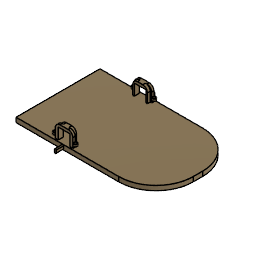
lab12 (Autodesk Fusion 360 design; units mm, degrees)
part number: 2026-05-18-18-22-44-675
Autodesk Fusion 360 part; units mm, degrees
sketch "sasiu" plane through (0, 0, 0) normal (0, 0, 1) x (1, 0, 0)
  line L0 (0, 0) -> (150, 0)
  line L1 (150, 0) -> (150, 90)
  line L2 (150, 90) -> (0, 90)
  line L3 (0, 90) -> (0, 0)
  line L4 (0, 0) -> (50, 0) construction
  line L5 (0, 0) -> (50, 0) construction
  line L6 (0, 90) -> (50, 90) construction
  line L7 (50, 0) -> (56.25, 0) construction
  line L8 (50, 0) -> (43.75, 0) construction
  line L9 (56.25, 0) -> (43.75, 0) construction
  line L10 (43.75, 0) -> (43.75, 24.2)
  line L11 (43.75, 24.2) -> (56.25, 24.2)
  line L12 (56.25, 24.2) -> (56.25, 0)
  line L13 (50, 90) -> (56.25, 90) construction
  line L14 (50, 90) -> (43.75, 90) construction
  line L15 (56.25, 90) -> (43.8642, 90) construction
  line L16 (43.8642, 90) -> (43.8642, 65.8)
  line L17 (43.8642, 65.8) -> (56.25, 65.8)
  line L18 (56.25, 65.8) -> (56.25, 90)
  line L19 (51, 0) -> (49, 0)
  line L20 (49, 0) -> (49, -7.85)
  line L21 (49, -7.85) -> (51, -7.85)
  line L22 (51, -7.85) -> (51, 0)
  line L23 (51, 90) -> (48.9753, 90)
  line L24 (48.9753, 90) -> (48.9753, 97.85)
  line L25 (48.9753, 97.85) -> (51, 97.85)
  line L26 (51, 97.85) -> (51, 90)
  line L27 (65.2982, 87.1869) -> (35.2982, 87.1869)
  line L28 (150, 45) -> (0, 45)
  line L29 (65.2982, 2.8131) -> (35.2982, 2.8131)
  line L30 (50, 90) -> (50, 0)
  circle A0 centre (60.9428, 87.1869) radius 2
  circle A1 centre (39.0572, 87.1869) radius 2
  circle A2 centre (60.9428, 2.8131) radius 2
  circle A3 centre (39.0572, 2.8131) radius 2
  circle A4 centre (60.9428, 87.1869) radius 1.25
  circle A5 centre (39.0572, 87.1869) radius 1.25
  circle A6 centre (60.9428, 2.8131) radius 1.25
  circle A7 centre (39.0572, 2.8131) radius 1.25
  line L31 (59.4051, 88.4658) -> (56.25, 88.4658)
  line L32 (56.25, 88.4658) -> (56.25, 85.9998)
  line L33 (56.25, 85.9998) -> (59.4051, 85.9998)
  line L34 (59.4051, 85.9998) -> (59.4051, 88.4658)
  line L35 (59.4051, 1.5342) -> (56.25, 1.5342)
  line L36 (59.4051, 4.0002) -> (59.4051, 1.5342)
  line L37 (56.25, 4.0002) -> (59.4051, 4.0002)
  line L38 (40.6669, 88.3739) -> (43.8642, 88.3739)
  line L39 (43.8642, 88.3739) -> (43.8642, 86)
  line L40 (43.8642, 86) -> (40.6669, 86)
  line L41 (40.6669, 86) -> (40.6669, 88.3739)
  line L42 (56.25, 88.4658) -> (43.8642, 88.4658)
  line L43 (57.8275, 85.9998) -> (57.8275, 83)
  line L44 (57.8275, 83) -> (42, 83)
  line L45 (42, 83) -> (42, 86)
  line L46 (57.8275, 7) -> (42, 7)
  line L47 (57.8275, 4.0002) -> (57.8275, 7)
  line L48 (42, 7) -> (42, 4)
  line L49 (43.75, 4.0002) -> (40.5949, 4.0002)
  line L50 (40.5949, 1.5342) -> (43.75, 1.5342)
  line L51 (40.5949, 4.0002) -> (40.5949, 1.5342)
  line L52 (56.25, 1.5342) -> (43.75, 1.5342)
  line L53 (57.8275, 85.9998) -> (57.8275, 88.4658)
  line L54 (42, 86) -> (42, 88.3739)
  line L55 (42, 4) -> (42, 1.5342)
  line L56 (57.8275, 4.0002) -> (57.8275, 1.5342)
  dimension "d1" = 150
  dimension "d2" = 90
  dimension "d3" = 50
  dimension "d4" = 50
  dimension "d5" = 6.25
  dimension "d6" = 6.25
  dimension "d7" = 24.2
  dimension "d8" = 6.25
  dimension "d9" = 6.25
  dimension "d10" = 24.2
  dimension "d11" = 7.85
  dimension "d12" = 7.85
  dimension "d13" = 43.8642
  dimension "d14" = 43.75
  dimension "d15" = 2
  dimension "d16" = 48.9753
  dimension "d17" = 2.0247
  dimension "d18" = 49
  dimension "d21" = 4
  dimension "d22" = 2.5
  dimension "d29" = 2.3739
  dimension "d30" = 3.1974
  dimension "d31" = 2.466
  dimension "d32" = 18.8102
  dimension "d33" = 15.8275
  dimension "d34" = 30
  dimension "d35" = 35.2982
  dimension "d36" = 86
  dimension "d37" = 83
  constraint horizontal L0
  constraint vertical L1
  constraint horizontal L2
  constraint vertical L3
  constraint coincident L0.start L3.end
  constraint coincident L0 L4.end
  constraint perpendicular L3 L5
  constraint perpendicular L3 L6
  constraint parallel L0 L7
  constraint parallel L0 L8
  constraint horizontal L9
  constraint vertical L10
  constraint horizontal L11
  constraint vertical L12
  constraint parallel L2 L13
  constraint parallel L6 L14
  constraint horizontal L15
  constraint vertical L16
  constraint horizontal L17
  constraint vertical L18
  constraint horizontal L19
  constraint vertical L20
  constraint horizontal L21
  constraint vertical L22
  constraint coincident L9 L19.start
  constraint horizontal L23
  constraint vertical L24
  constraint horizontal L25
  constraint vertical L26
  constraint coincident L2 L23.start
  constraint perpendicular L16 L27
  constraint midpoint L1 L28.start
  constraint midpoint L3 L28.end
  constraint symmetric L27.start L28 L29.start
  constraint symmetric L27.end L28 L29.end
  constraint perpendicular L4 L30
  constraint coincident L27 A0.centre
  constraint symmetric L30 A0 A1
  constraint symmetric L28 A0 A2
  constraint symmetric L28 A1 A3
  constraint concentric A0 A4
  constraint symmetric L30 A4 A5
  constraint symmetric L28 A4 A6
  constraint symmetric L28 A5 A7
  constraint horizontal L31
  constraint vertical L32
  constraint horizontal L33
  constraint vertical L34
  constraint coincident L18 L32.end
  constraint coincident A0 L31.start
  constraint symmetric L28 L31.start L35.start
  constraint symmetric L28 L31.end L35.end
  constraint symmetric L28 L32.end L37.start
  constraint symmetric L28 L33.end L36.start
  constraint horizontal L38
  constraint vertical L39
  constraint horizontal L40
  constraint vertical L41
  constraint coincident L16 L39.end
  constraint coincident A1 L38.start
  constraint coincident A1 L40.end
  constraint coincident L16 L42.end
  constraint perpendicular L16 L42
  constraint midpoint L33 L43.start
  constraint perpendicular L33 L43
  constraint perpendicular L16 L44
  constraint coincident L40 L45.end
  constraint perpendicular L40 L45
  constraint symmetric L28 L43.start L47.start
  constraint symmetric L28 L43.end L46.start
  constraint symmetric L28 L44.end L46.end
  constraint symmetric L28 L45.end L48.end
  constraint symmetric L30 L35.start L50.start
  constraint symmetric L30 L35.end L50.end
  constraint symmetric L30 L36.start L49.end
  constraint symmetric L30 L37.start L49.start
  constraint midpoint L31 L53.end
  constraint coincident L38 L54.end
  constraint perpendicular L38 L54
  constraint coincident L50 L55.end
  constraint perpendicular L50 L55
  constraint midpoint L35 L56.end
  measures "d1" distance of L0.start L0.end
  measures "d2" distance of L0.start L2.end
  measures "d3" distance of L0.start L4.end
  measures "d4" distance of L2.end L6.end
  measures "d5" distance of L4.end L7.end
  measures "d6" distance of L4.end L8.end
  measures "d7" distance of L7.end L11.end
  measures "d8" distance of L6.end L13.end
  measures "d9" distance of L6.end L14.end
  measures "d10" distance of L13.end L17.end
  measures "d11" distance of L19.start L21.end
  measures "d12" distance of L23.start L25.end
  measures "d13" distance of L3 L16
  measures "d14" distance of L3 L10
  measures "d15" distance of L20 L22
  measures "d16" distance of L3 L24
  measures "d17" distance of L24 L26
  measures "d18" distance of L3 L20
  measures "d21" diameter of A0
  measures "d22" diameter of A4
  measures "d29" distance of L38 L40
  measures "d30" distance of L39 L41
  measures "d31" distance of L33 L42
  measures "d32" distance of L34 L51
  measures "d33" distance of L53 L54
  measures "d34" horizontal distance of L29.start L29.end
  measures "d35" distance of L3 L27.end
  measures "d36" distance of L0 L40
  measures "d37" distance of L0 L44
extrude "Extrude1" add sketch "sasiu" along normal blind 5 makes body 1
extrude "Extrude2" add sketch "sasiu" along normal blind 2 from surface at 8 separate body contours L29 A3 A7 L51 | L29 A3 A7 L49 L51 | L29 A2 A6 L36 | L29 A2 A6 L36 L37 | L27 A1 A5 L41 | L27 A1 A5 L41 | L27 A0 A4 L34 | L27 A0 A4 L33 L34 makes body 2 at (60.1621, 4.6544, 8.6667) makes body 3 at (38.8689, 0.8219, 8.6667) makes body 4 at (62.738, 88.0687, 9.3333) makes body 5 at (40.5426, 85.8478, 8.6667)
extrude "Extrude3" add sketch "sasiu" along normal blind 15 from surface at 5 contours L10 L29 L50 L55 | L10 L29 L49 L55 | L29 A3 L50 L55 | L10 L46 L48 L49 | L29 A3 L49 L55 | L29 A3 L51 | L12 L29 L35 L56 | L12 L29 L37 L56 | L29 A3 L49 L51 | L29 A2 L35 L56 | L16 L27 L38 L39 L54 | L16 L40 L44 L45 | L18 L33 L43 L44 | L12 L37 L46 L47 | L29 A2 L37 L56 | L29 A2 L36 | L16 L27 L39 L40 L54 | L27 A1 L38 L54 | L18 L27 L31 L32 L53 | L18 L27 L32 L33 L53 | L29 A2 L36 L37 | L27 A1 L40 L54 | L27 A1 L41 | L27 A0 L31 L53 | L27 A0 L33 L53 | L27 A1 L41 | L27 A0 L34 | L27 A0 L33 L34 bodies 2 3 4 5
combine "Combine1" operation add target body 1 tool bodies 2 3 4 5
extrude "Extrude5" add sketch "sasiu" along normal blind 3 from surface at 17 contours L10 L29 L50 L55 | L10 L29 L30 L52 | L10 L29 L49 L55 | L10 L29 L30 L46 | L12 L29 L30 L52 | L10 L46 L48 L49 | L12 L29 L30 L46 | L12 L29 L35 L56 | L16 L27 L30 L39 L42 | L16 L27 L30 L39 L44 | L18 L27 L30 L32 L44 | L12 L29 L37 L56 | L16 L27 L38 L39 L54 | L18 L27 L30 L32 L42 | L16 L40 L44 L45 | L18 L33 L43 L44 | L12 L37 L46 L47 | L16 L27 L39 L40 L54 | L18 L27 L31 L32 L53 | L18 L27 L32 L33 L53 bodies 1
fillet "Fillet1" radius 40 2 edges at (150, 0, 2.5) (150, 90, 2.5) on bodies 1
fillet "Fillet2" radius 1 4 edges at (51, 93.925, 5) (51, 93.925, 0) (48.9753, 93.925, 5) (48.9753, 93.925, 0) on bodies 1
fillet "Fillet3" radius 1 4 edges at (49, -3.925, 5) (49, -3.925, 0) (51, -3.925, 5) (51, -3.925, 0) on bodies 1
fillet "Fillet4" radius 5 4 edges at (40.6669, 87.1869, 20) (42, 84.5, 20) (57.8275, 84.4999, 20) (59.4051, 87.2328, 20) on bodies 1
fillet "Fillet5" radius 5 4 edges at (59.4051, 2.7672, 20) (57.8275, 5.5001, 20) (42, 5.5001, 20) (40.5949, 2.7672, 20) on bodies 1
named bodies: "sasiu"
